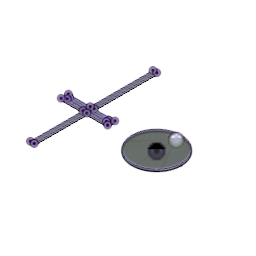
basic scotch yoke components (Autodesk Fusion 360 design; units mm, degrees)
part number: 2026-07-02-11-30-03-553
Autodesk Fusion 360 part; units mm, degrees
sketch "Sketch1" plane through (0, 0, 0) normal (0, 0, 1) x (1, 0, 0)
  line L0 (-134.9268, 7.45) -> (-134.9268, 135.2463)
  line L1 (-99.95, -2.45) -> (-99.95, -2.4)
  line L2 (-187.45, 7.45) -> (-187.45, -7.45)
  line L3 (-134.9268, 135.2463) -> (-142.9268, 135.2463)
  line L4 (-134.9268, -7.45) -> (-92.55, -7.45)
  line L5 (-99.95, 2.45) -> (-180.05, 2.45)
  line L6 (-92.55, -7.45) -> (-92.55, 7.45)
  arc A0 (-99.95, -2.45) -> (-99.95, 2.45) centre (-99.95, 0) ccw
  line L7 (-134.9268, -114.7537) -> (-134.9268, -7.45)
  line L8 (-99.95, 2.4) -> (-99.95, 2.45)
  line L9 (-180.05, -2.45) -> (-99.95, -2.45)
  line L10 (-92.55, 7.45) -> (-134.9268, 7.45)
  line L11 (-142.9268, 7.45) -> (-187.45, 7.45)
  arc A1 (-180.05, 2.45) -> (-180.05, -2.45) centre (-180.05, 0) ccw
  line L12 (-142.9268, 135.2463) -> (-142.9268, 7.45)
  line L13 (-142.9268, -7.45) -> (-142.9268, -114.7537)
  line L14 (-142.9268, -114.7537) -> (-134.9268, -114.7537)
  line L15 (-187.45, -7.45) -> (-142.9268, -7.45)
  point P0 (-140, 0)
  point P1 (-99.95, 0)
  point P2 (-180.05, 0)
  point P3 (-140, 0)
  point P4 (-140, 0)
  point P5 (-140, 0)
  dimension "d12" = 8
  dimension "d13" = 250
  dimension "d14" = 94.9
  dimension "d15" = 14.9
  dimension "d16" = 80.1
  dimension "d17" = 4.9
  dimension "d18" = 4.9
  dimension "d19" = 4.9
  constraint horizontal L3
  constraint perpendicular L3 L12
  constraint parallel L3 L14
  constraint parallel L0 L12
  constraint coincident P5 P4
  constraint horizontal L10
  constraint perpendicular L2 L11
  constraint parallel L4 L10
  constraint parallel L2 L6
  constraint horizontal L5
  constraint parallel L5 L9
  constraint collinear L1 L8
  constraint coincident P1 L1
  constraint coincident P1 A0.centre
  constraint coincident P2 A1.centre
  constraint collinear L12 L13
  constraint collinear L0 L7
  constraint collinear L10 L11
  constraint collinear L4 L15
  measures "d12" distance of L13.end L7.start
  measures "d13" distance of L13.end L3.end
  measures "d14" distance of L4.end L2.end
  measures "d15" distance of L2.start L2.end
  measures "d16" distance of L1.start L9.start
  measures "d17" distance of L9.start L5.end
  measures "d18" diameter of A0
  measures "d19" diameter of A1
sketch "Sketch2" plane through (0, 0, 0) normal (0, 0, 1) x (1, 0, 0)
  circle A0 centre (0, 0) radius 50
  circle A1 centre (0, 40) radius 2.4
  dimension "d20" = 100
  dimension "d22" = 4.8
  constraint coincident A0.centre origin
  measures "d20" diameter of A0
  measures "d22" diameter of A1
extrude "Extrude1" add sketch "Sketch2" along normal blind 4 makes body 1
extrude "Extrude2" add sketch "Sketch1" along normal blind 4 separate body makes body 2
sketch "Sketch5" plane through (0, 0, 4) normal (0, 0, 1) x (-1, 0, 0)
  circle A0 centre (0, -40) radius 2.4
  circle A1 centre (0, 0) radius 50
  arc A2 (180.05, -2.45) -> (180.05, 2.45) centre (180.05, 0) ccw
  line L0 (180.05, -2.45) -> (99.95, -2.45)
  arc A3 (99.95, 2.45) -> (99.95, -2.45) centre (99.95, 0) ccw
  line L1 (99.95, 2.45) -> (180.05, 2.45)
  line L2 (187.45, 7.45) -> (142.9268, 7.45)
  line L3 (142.9268, 7.45) -> (142.9268, 114.7537)
  line L4 (142.9268, 114.7537) -> (134.9268, 114.7537)
  line L5 (134.9268, 114.7537) -> (134.9268, 7.45)
  line L6 (134.9268, 7.45) -> (92.55, 7.45)
  line L7 (92.55, 7.45) -> (92.55, -7.45)
  line L8 (92.55, -7.45) -> (134.9268, -7.45)
  line L9 (134.9268, -7.45) -> (134.9268, -135.2463)
  line L10 (134.9268, -135.2463) -> (142.9268, -135.2463)
  line L11 (142.9268, -135.2463) -> (142.9268, -7.45)
  line L12 (142.9268, -7.45) -> (187.45, -7.45)
  line L13 (187.45, -7.45) -> (187.45, 7.45)
sketch "Sketch6" plane through (0, 0, 0) normal (0, 0, 1) x (1, 0, 0)
equation "d14 = ( 2 * 45 ) * 1 mm + 4.8 mm + 0.1 mm"
equation "d15 = ( 2 * 5 ) * 1 mm + 4.8 mm + 0.1 mm"
equation "d16 = ( 40 * 2 ) * 1 mm + 0.1 mm"
equation "d17 = 4.8 mm + 0.1 mm"
equation "d18 = 4.8 mm + 0.1 mm"
equation "d19 = 4.8 mm + 0.1 mm"
